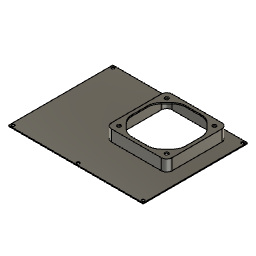
M2000 GPU Enclosure Lid v2 (Autodesk Fusion 360 design; units mm, degrees)
Autodesk Fusion 360 part; units mm, degrees
sketch "Sketch1" plane through (0, 0, 0) normal (0, 0, 1) x (1, 0, 0)
  line L0 (0, 0) -> (200, 0)
  line L1 (200, 0) -> (200, 155)
  line L2 (200, 155) -> (0, 155)
  line L3 (0, 155) -> (0, 0)
  line L4 (135, 100) -> (135, 145) construction
  line L5 (135, 100) -> (135, 55) construction
  circle A0 centre (135, 100) radius 40 construction
  line L6 (135, 100) -> (90, 100) construction
  line L7 (135, 100) -> (180, 100) construction
  line L8 (90, 145) -> (180, 145) construction
  line L9 (180, 145) -> (180, 55) construction
  line L10 (180, 55) -> (90, 55) construction
  line L11 (90, 55) -> (90, 145) construction
  line L12 (90, 145) -> (92.4, 145) construction
  line L13 (92.4, 145) -> (92.4, 142.6) construction
  line L14 (92.4, 142.6) -> (90, 142.6) construction
  line L15 (90, 142.6) -> (90, 145) construction
  line L16 (180, 55) -> (177.6, 55) construction
  line L17 (177.6, 55) -> (177.6, 57.4) construction
  line L18 (177.6, 57.4) -> (180, 57.4) construction
  line L19 (180, 57.4) -> (180, 55) construction
  line L20 (90, 145) -> (180, 145)
  line L21 (180, 145) -> (180, 55)
  line L22 (180, 55) -> (90, 55)
  line L23 (90, 55) -> (90, 145)
  line L24 (92.4, 142.6) -> (177.6, 142.6)
  line L25 (177.6, 142.6) -> (177.6, 57.4)
  line L26 (177.6, 57.4) -> (92.4, 57.4)
  line L27 (92.4, 57.4) -> (92.4, 142.6)
  dimension "d1" = 200
  dimension "d2" = 155
  dimension "d5" = 2.4
  dimension "d6" = 2.4
  dimension "d7" = 2.4
  dimension "d8" = 2.4
  constraint horizontal L0
  constraint vertical L1
  constraint horizontal L2
  constraint vertical L3
  constraint coincident L0.start L3.end
  constraint coincident L4.start L5.start
  constraint perpendicular L5 L6
  constraint perpendicular L4 L7
  constraint horizontal L8
  constraint vertical L9
  constraint horizontal L10
  constraint vertical L11
  constraint horizontal L12
  constraint vertical L13
  constraint horizontal L14
  constraint vertical L15
  constraint horizontal L16
  constraint vertical L17
  constraint horizontal L18
  constraint vertical L19
  constraint horizontal L20
  constraint vertical L21
  constraint horizontal L22
  constraint vertical L23
  constraint horizontal L24
  constraint vertical L25
  constraint horizontal L26
  constraint vertical L27
  measures "d1" distance of L0.start L0.end
  measures "d2" distance of L0.start L2.end
  measures "d5" distance of L8.start L12.end
  measures "d6" distance of L8.start L14.end
  measures "d7" distance of L9.end L16.end
  measures "d8" distance of L9.end L18.end
extrude "Extrude1" add sketch "Sketch1" against normal blind 1.2 contours L0 L1 L2 L3 makes body 1
extrude "Extrude2" add sketch "Sketch1" along normal blind 15 separate body contours L20 L21 L22 L23 makes body 2
sketch "Sketch2" plane through (0, 0, 15) normal (0, 0, 1) x (-1, 0, 0)
  line L0 (-177.6, -57.4) -> (-92.4, -57.4)
  line L1 (-92.4, -57.4) -> (-92.4, -142.6)
  line L2 (-92.4, -142.6) -> (-177.6, -142.6)
  line L3 (-177.6, -142.6) -> (-177.6, -57.4)
  line L4 (-90, -55) -> (-180, -55)
  line L5 (-180, -55) -> (-180, -145)
  line L6 (-180, -145) -> (-90, -145)
  line L7 (-90, -145) -> (-90, -55)
  line L8 (-95, -140) -> (-99.5, -140) construction
  line L9 (-99.5, -140) -> (-99.5, -135.5) construction
  line L10 (-99.5, -135.5) -> (-95, -135.5) construction
  line L11 (-95, -135.5) -> (-95, -140) construction
  line L12 (-175, -60) -> (-170.5, -60) construction
  line L13 (-170.5, -60) -> (-170.5, -64.5) construction
  line L14 (-170.5, -64.5) -> (-175, -64.5) construction
  line L15 (-175, -64.5) -> (-175, -60) construction
  line L16 (-99.5, -135.5) -> (-170.5, -135.5) construction
  line L17 (-170.5, -135.5) -> (-170.5, -64.5) construction
  line L18 (-170.5, -64.5) -> (-99.5, -64.5) construction
  line L19 (-99.5, -64.5) -> (-99.5, -135.5) construction
  circle A0 centre (-99.5, -135.5) radius 2.75
  circle A1 centre (-170.5, -135.5) radius 2.75
  circle A2 centre (-99.5, -64.5) radius 2.75
  circle A3 centre (-170.5, -64.5) radius 2.75
  line L20 (-115, -140) -> (-95, -120)
  line L21 (-95, -120) -> (-95, -80)
  line L22 (-95, -80) -> (-115, -60)
  line L23 (-115, -60) -> (-155, -60)
  line L24 (-155, -60) -> (-175, -80)
  line L25 (-175, -80) -> (-175, -120)
  line L26 (-175, -120) -> (-155, -140)
  line L27 (-155, -140) -> (-115, -140)
  line L28 (-90, -145) -> (-180, -145)
  line L29 (-180, -145) -> (-180, -55)
  line L30 (-180, -55) -> (-90, -55)
  line L31 (-90, -55) -> (-90, -145)
  dimension "d13" = 4.5
  dimension "d14" = 4.5
  dimension "d15" = 4.5
  dimension "d16" = 4.5
  dimension "d17" = 5.5
  dimension "d18" = 5.5
  dimension "d19" = 5.5
  dimension "d20" = 5.5
  constraint horizontal L8
  constraint vertical L9
  constraint horizontal L10
  constraint vertical L11
  constraint horizontal L12
  constraint vertical L13
  constraint horizontal L14
  constraint vertical L15
  constraint horizontal L16
  constraint vertical L17
  constraint horizontal L18
  constraint vertical L19
  constraint coincident L9.end L10.start
  constraint coincident L16.end L17.start
  constraint coincident L18.end L19.start
  constraint coincident L13.end L14.start
  constraint parallel L1 L21
  constraint perpendicular L21 L23
  constraint perpendicular L18 L25
  constraint perpendicular L24 L26
  constraint parallel L16 L27
  constraint horizontal L28
  constraint vertical L29
  constraint horizontal L30
  constraint vertical L31
  constraint coincident L4.end L5.start
  constraint coincident L6.end L7.start
  measures "d13" distance of L8.start L8.end
  measures "d14" distance of L8.start L10.end
  measures "d15" distance of L12.start L12.end
  measures "d16" distance of L12.start L14.end
  measures "d17" diameter of A0
  measures "d18" diameter of A1
  measures "d19" diameter of A2
  measures "d20" diameter of A3
extrude "Extrude3" add sketch "Sketch2" along normal blind 1.8 contours L0 L1 L2 L3 | L4 L5 L6 L7 L28 L29 L30 L31 bodies 2
fillet "Fillet1" radius 20 8 edges at (95, 80, 15.9) (115, 60, 15.9) (155, 60, 15.9) (175, 80, 15.9) (175, 120, 15.9) (155, 140, 15.9) (115, 140, 15.9) (95, 120, 15.9) on bodies 2
sketch "Sketch3" plane through (0, 0, 0) normal (0, 0, 1) x (1, 0, 0)
extrude "Extrude4" add sketch "Sketch1" against normal blind 1.2 contours L20 L21 L22 L23 bodies 1 2
fillet "Fillet2" radius 8 4 edges at (92.4, 142.6, 6.9) (177.6, 142.6, 6.9) (177.6, 57.4, 6.9) (92.4, 57.4, 6.9) on bodies 1
fillet "Fillet3" radius 8 4 edges at (90, 145, 8.4) (90, 55, 8.4) (180, 55, 8.4) (180, 145, 8.4) on bodies 1
sketch "Sketch4" plane through (0, 0, 0) normal (0, 0, 1) x (1, 0, 0)
  line L0 (200, 155) -> (196.5, 155) construction
  line L1 (196.5, 155) -> (196.5, 151.5) construction
  line L2 (196.5, 151.5) -> (200, 151.5) construction
  line L3 (200, 151.5) -> (200, 155) construction
  line L4 (0, 0) -> (3.5, 0) construction
  line L5 (3.5, 0) -> (3.5, 3.5) construction
  line L6 (3.5, 3.5) -> (0, 3.5) construction
  line L7 (0, 3.5) -> (0, 0) construction
  line L8 (3.5, 3.5) -> (196.5, 3.5) construction
  line L9 (196.5, 3.5) -> (196.5, 151.5) construction
  line L10 (196.5, 151.5) -> (3.5, 151.5) construction
  line L11 (3.5, 151.5) -> (3.5, 3.5) construction
  circle A0 centre (3.5, 151.5) radius 2.15
  circle A1 centre (3.5, 3.5) radius 2.15
  circle A2 centre (196.5, 151.5) radius 2.15
  circle A3 centre (196.5, 3.5) radius 2.15
  circle A4 centre (79.8779, 151.5) radius 2.1
  circle A5 centre (100, 3.5) radius 2.1
  dimension "d31" = 3.5
  dimension "d32" = 3.5
  dimension "d33" = 3.5
  dimension "d34" = 3.5
  dimension "d35" = 4.3
  dimension "d36" = 4.3
  dimension "d37" = 4.3
  dimension "d38" = 4.3
  dimension "d41" = 4.2
  dimension "d42" = 4.2
  constraint horizontal L0
  constraint vertical L1
  constraint horizontal L2
  constraint vertical L3
  constraint horizontal L4
  constraint vertical L5
  constraint horizontal L6
  constraint vertical L7
  constraint coincident L4.start L7.end
  constraint horizontal L8
  constraint vertical L9
  constraint horizontal L10
  constraint vertical L11
  constraint coincident L10.end L11.start
  constraint coincident L5.end L6.start
  constraint coincident L1.end L2.start
  constraint coincident L8.end L9.start
  constraint coincident L10 A4.centre
  constraint midpoint L8 A5.centre
  measures "d31" distance of L0.start L0.end
  measures "d32" distance of L0.start L2.end
  measures "d33" distance of L4.start L4.end
  measures "d34" distance of L4.start L6.end
  measures "d35" diameter of A0
  measures "d36" diameter of A1
  measures "d37" diameter of A2
  measures "d38" diameter of A3
  measures "d41" diameter of A4
  measures "d42" diameter of A5
extrude "Extrude5" cut sketch "Sketch4" against normal blind 1.2 contours A0 | A1 | A2 | A3 bodies 1
extrude "Extrude6" cut sketch "Sketch4" against normal blind 1.2 contours A4 | A5 bodies 1
copy_body "Body->Comp1" bodies 1 removing the originals makes body 3 in component "Component"
component "Component" placed x (1, 0, 0) y (0, 1, 0) z (0, 0, 1) at (0, 0, 0)
